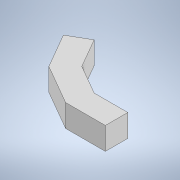
# Autodesk Inventor part: finger_two_bend
Saved by Autodesk Inventor 2021 (Build 250183000, 183)
## iProperties
Created: 2021-03-11
Part Number: finger_two_bend
Material: Generic
Document SubType Name: Modeling
Designer: Charlie
Density: 1 g/cm^3
Appearance: Default
Author: Charlie
Autodesk Inventor part; units mm, degrees
ref_plane "YZ Plane" through (0, 0, 0) normal (1, 0, 0) x (0, 1, 0)
ref_plane "XZ Plane" through (0, 0, 0) normal (0, 1, 0) x (-1, 0, 0)
ref_plane "XY Plane" through (0, 0, 0) normal (0, 0, 1) x (1, 0, 0)
sketch "Sketch1" plane through (0, 0, 0) normal (0, 1, 0) x (-1, 0, 0)
  line L0 (-15, 10) -> (20.359, 10)
  line L1 (25, 7.3205) -> (15, -10) construction
  line L2 (15, -10) -> (-15, -10)
  line L3 (-15, -10) -> (-15, 10)
  line L4 (-15, 10) -> (15, -10) construction
  line L5 (15, 10) -> (-15, -10) construction
  line L6 (20.359, 10) -> (55.6218, -10.359)
  line L7 (58.3013, -15) -> (40.9808, -25) construction
  line L8 (40.9808, -25) -> (15, -10)
  line L9 (15, -10) -> (15, 10) construction
  line L10 (55.6218, -10.359) -> (73.3013, -40.9808)
  line L11 (73.3013, -40.9808) -> (55.9808, -50.9808)
  line L12 (55.9808, -50.9808) -> (40.9808, -25)
  line L13 (40.9808, -25) -> (50.9808, -7.6795) construction
  point P0 (0, 0)
  point P1 (15, -10)
  dimension "d0" = 30
  constraints: 28 end point, 3 parallel, 2 midpoint, 2 point on line, 1 horizontal, 1 perpendicular
  measures "d0" distance of L2.start L2.end
extrude "Extrusion1" add sketch "Sketch1" along normal blind 20
body "Solid1"
